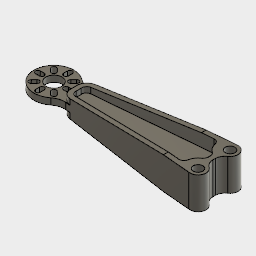
C04-W1-LC-01 (Autodesk Fusion 360 design; units mm, degrees)
Autodesk Fusion 360 part; units mm, degrees
sketch "Layout Sketch" plane through (0, 0, 0) normal (0, 1, 0) x (1, 0, 0)
  circle A0 centre (0, 0) radius 5
  circle A1 centre (0, 0) radius 12.5
  line L0 (-1.5, 10) -> (-1.5, 7.5)
  arc A2 (-1.5, 7.5) -> (1.5, 7.5) centre (0, 7.5) ccw
  line L1 (1.5, 7.5) -> (1.5, 10)
  arc A3 (1.5, 10) -> (-1.5, 10) centre (0, 10) ccw
  line L2 (0, 10) -> (0, 7.5) construction
  arc A4 (-6.0104, 8.1317) -> (-8.1317, 6.0104) centre (-7.0711, 7.0711) ccw
  line L3 (-8.1317, 6.0104) -> (-6.364, 4.2426)
  arc A5 (-6.364, 4.2426) -> (-4.2426, 6.364) centre (-5.3033, 5.3033) ccw
  line L4 (-4.2426, 6.364) -> (-6.0104, 8.1317)
  arc A6 (-10, 1.5) -> (-10, -1.5) centre (-10, 0) ccw
  line L5 (-10, -1.5) -> (-7.5, -1.5)
  arc A7 (-7.5, -1.5) -> (-7.5, 1.5) centre (-7.5, 0) ccw
  line L6 (-7.5, 1.5) -> (-10, 1.5)
  arc A8 (-8.1317, -6.0104) -> (-6.0104, -8.1317) centre (-7.0711, -7.0711) ccw
  line L7 (-6.0104, -8.1317) -> (-4.2426, -6.364)
  arc A9 (-4.2426, -6.364) -> (-6.364, -4.2426) centre (-5.3033, -5.3033) ccw
  line L8 (-6.364, -4.2426) -> (-8.1317, -6.0104)
  arc A10 (-1.5, -10) -> (1.5, -10) centre (0, -10) ccw
  line L9 (1.5, -10) -> (1.5, -7.5)
  arc A11 (1.5, -7.5) -> (-1.5, -7.5) centre (0, -7.5) ccw
  line L10 (-1.5, -7.5) -> (-1.5, -10)
  arc A12 (6.0104, -8.1317) -> (8.1317, -6.0104) centre (7.0711, -7.0711) ccw
  line L11 (8.1317, -6.0104) -> (6.364, -4.2426)
  arc A13 (6.364, -4.2426) -> (4.2426, -6.364) centre (5.3033, -5.3033) ccw
  line L12 (4.2426, -6.364) -> (6.0104, -8.1317)
  arc A14 (10, -1.5) -> (10, 1.5) centre (10, 0) ccw
  line L13 (10, 1.5) -> (7.5, 1.5)
  arc A15 (7.5, 1.5) -> (7.5, -1.5) centre (7.5, 0) ccw
  line L14 (7.5, -1.5) -> (10, -1.5)
  arc A16 (8.1317, 6.0104) -> (6.0104, 8.1317) centre (7.0711, 7.0711) ccw
  line L15 (6.0104, 8.1317) -> (4.2426, 6.364)
  arc A17 (4.2426, 6.364) -> (6.364, 4.2426) centre (5.3033, 5.3033) ccw
  line L16 (6.364, 4.2426) -> (8.1317, 6.0104)
  line L17 (0, 0) -> (100, 0) construction
  line L18 (100, 15) -> (100, -15)
  line L19 (100, 15) -> (10.2544, 7.1483)
  line L20 (10.2544, -7.1483) -> (100, -15)
  circle A18 centre (100, 10) radius 5
  circle A19 centre (100, -10) radius 5
  dimension "d1" = 10
  dimension "d2" = 25
  dimension "d3" = 3
  dimension "d4" = 10
  dimension "d5" = 7.5
  dimension "d7" = 360
  dimension "d18" = 100
  dimension "d19" = 30
  dimension "d20" = 5
  dimension "d21" = 5
  dimension "d22" = 10
  measures "d1" diameter of A0
  measures "d2" diameter of A1
  measures "d3" diameter of A2
  measures "d4" distance of A0.centre A3.centre
  measures "d5" distance of A0.centre A2.centre
  measures "d18" distance of A0.centre L17.end
  measures "d19" distance of L18.start L18.end
  measures "d20" angle of L17 L20
  measures "d21" angle of L17 L19
  measures "d22" diameter of A18
extrude "Extrude1" add sketch "Layout Sketch" along normal mid plane 4 contours A1 | A1 L18 L19 L20 A18 A19 | L18 L19 A18 | L18 L20 A19 | L18 A18 | L18 A19 makes body 1
sketch "Mounting Point" plane through (0, 0, 0) normal (0, 1, 0) x (1, 0, 0)
  circle A0 centre (100, 10) radius 3
  circle A1 centre (100, -10) radius 3
  circle A2 centre (100, 10) radius 5
  circle A3 centre (100, -10) radius 5
  point P0 (100, 10)
  point P1 (100, -10)
  dimension "d23" = 6
  measures "d23" diameter of A1
extrude "Extrude2" add sketch "Mounting Point" along normal mid plane 20 bodies 1
extrude "Extrude3" add sketch "Layout Sketch" along normal blind 10 separate body contours A1 L18 L19 L20 A18 A19 makes body 2
sketch "Profile Cut" plane through (0, 0, 0) normal (0, 0, 1) x (1, 0, 0)
  line L0 (10.2544, 10) -> (99.1318, 10)
  line L1 (99.1318, 10) -> (10.2544, 10)
  line L2 (99.1318, 10) -> (81.7577, 10)
  line L3 (10.2544, 0) -> (10.2544, 10)
  line L4 (81.7577, 10) -> (10.2544, 5)
  line L5 (10.2544, 5) -> (10.2544, 0)
  line L6 (99.1318, 10) -> (99.1318, 0)
  point P0 (99.1318, 10)
  point P1 (99.1318, 10)
  point P2 (99.1318, 0)
  dimension "d28" = 4
  measures "d28" angle of L0 L4
split "Split1" by curves path "Profile Cut" along L2 L4 L5 bodies 2 makes body 3 at (58.6718, 10, 0)
delete_body "RemoveBody1" bodies 3
sketch "Wall thickness" plane through (0, 0, 0) normal (0, 1, 0) x (1, 0, 0)
  line L0 (100, 15) -> (10.2544, 7.1483)
  line L1 (10.2544, -7.1483) -> (100, -15)
  circle A0 centre (0, 0) radius 12.5
  circle A1 centre (100, 10) radius 5
  circle A2 centre (100, -10) radius 5
  line L2 (100, 15) -> (100, -15)
  line L3 (10.5158, -4.1597) -> (97, -11.7261)
  line L4 (97, 11.7261) -> (97, -11.7261)
  line L5 (97, 11.7261) -> (10.5158, 4.1597)
  circle A3 centre (100, 10) radius 8
  circle A4 centre (100, -10) radius 8
  circle A5 centre (0, 0) radius 15.5
  dimension "d29" = 3
  dimension "d30" = 3
  dimension "d31" = 3
  dimension "d32" = 3
extrude "Extrude4" cut sketch "Wall thickness" along normal blind 15 contours L3 L4 L5 A3 A4 A5 bodies 2
mirror "Mirror1" about plane through (0, 0, 0) normal (0, 1, 0) of bodies 2 makes body 4
combine "Combine1" operation add target body 2 tool bodies 4 1
fillet "Fillet1" radius 3 12 edges at (92.106, 6, -11.2979) (97, 6, -2.5838) (97, 6, 2.5838) (92.106, 6, 11.2979) (14.8213, 3.6597, -4.5364) (14.8213, 3.6597, 4.5364) (92.106, -6, 11.2979) (97, -6, 2.5838) (97, -6, -2.5838) (92.106, -6, -11.2979) (14.8213, -3.6597, -4.5364) (14.8213, -3.6597, 4.5364) on bodies 2
fillet "Fillet2" radius 6 6 edges at (100, 0, -5) (100, 0, 5) (10.2544, 3.5, -7.1483) (10.2544, 3.5, 7.1483) (10.2544, -3.5, 7.1483) (10.2544, -3.5, -7.1483) on bodies 2
fillet "Fillet3" radius 10 2 edges at (10.2544, 0, 7.1483) (10.2544, 0, -7.1483) on bodies 2
equation "d30 = d29"
equation "d31 = d29"
equation "d32 = d29"
